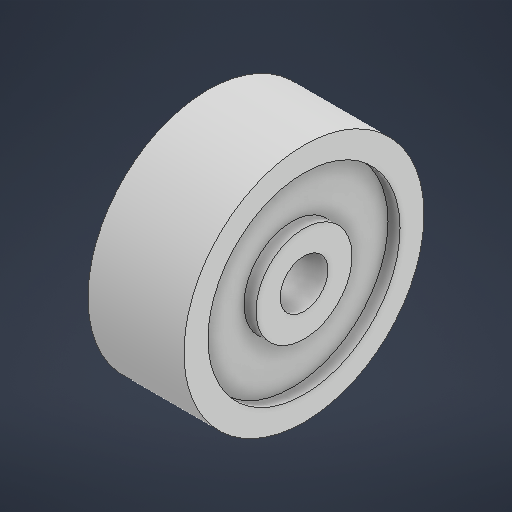
# Autodesk Inventor part: Peça1
Saved by Autodesk Inventor 2027 (Build 310192060, 192F)
## iProperties
Created: 2026-08-25
Part Number: Peça1
Material: Genérico
Document SubType Name: Modeling
Designer: guisg
Density: 1 g/cm^3
Appearance: Padrão
Author: guisg
Autodesk Inventor part; units mm, degrees
ref_plane "YZ Plane" through (0, 0, 0) normal (1, 0, 0) x (0, 1, 0)
ref_plane "XZ Plane" through (0, 0, 0) normal (0, 1, 0) x (-1, 0, 0)
ref_plane "XY Plane" through (0, 0, 0) normal (0, 0, 1) x (1, 0, 0)
sketch "Esboço1" plane through (0, 0, 0) normal (1, 0, 0) x (0, 1, 0)
  circle A0 centre (0, 0) radius 50
  circle A1 centre (0, 0) radius 40
  circle A2 centre (0, 0) radius 10
  circle A3 centre (0, 0) radius 20
  constraints: 4 centre point, 4 coincident
extrude "Extrusão1" add sketch "Esboço1" along normal mid plane 40
sketch "Esboço3" plane through (0, 0, 0) normal (1, 0, 0) x (0, 1, 0)
  circle A0 centre (0, 0) radius 20
  circle A1 centre (0, 0) radius 40
  constraints: 2 centre point, 2 coincident
extrude "Extrusão2" add sketch "Esboço3" along normal mid plane 30
